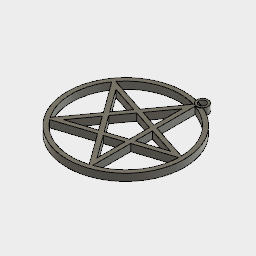
五角星挂件 v0 (Autodesk Fusion 360 design; units mm, degrees)
Autodesk Fusion 360 part; units mm, degrees
sketch "草图1" plane through (0, 0, 0) normal (0, 1, 0) x (1, 0, 0)
  circle A0 centre (70, -20) radius 40.6099
  line L0 (80.6872, 16.0595) -> (65.2067, -5.2476)
  line L1 (79.5492, 9.3893) -> (68.2067, -6.2223)
  line L2 (40.1586, 2.891) -> (65.2067, -5.2476)
  line L3 (45, -1.8364) -> (63.3525, -7.7995)
  line L4 (45, -1.8364) -> (56.3425, -17.448)
  line L5 (63.3525, -7.7995) -> (56.3425, -17.448)
  line L6 (54.4884, -20) -> (39.0079, -41.3071)
  line L7 (66.3525, -8.7743) -> (58.1966, -20)
  line L8 (56.3425, -22.552) -> (45, -38.1636)
  line L9 (39.0079, 1.3071) -> (54.4884, -20)
  line L10 (65.2067, -34.7524) -> (40.1586, -42.891)
  line L11 (56.3425, -22.552) -> (63.3525, -32.2005)
  line L12 (65.2067, -34.7524) -> (80.6872, -56.0595)
  line L13 (58.1966, -20) -> (66.3525, -31.2257)
  line L14 (68.2067, -33.7777) -> (79.5492, -49.3893)
  line L15 (63.3525, -32.2005) -> (45, -38.1636)
  line L16 (82.5492, -29.1175) -> (82.5492, -55.4545)
  line L17 (107.5972, -20.9789) -> (82.5492, -29.1175)
  line L18 (79.5492, -30.0923) -> (68.2067, -33.7777)
  line L19 (79.5492, -30.0923) -> (79.5492, -49.3893)
  line L20 (100.9017, -20) -> (82.5492, -25.9631)
  line L21 (79.5492, -26.9379) -> (66.3525, -31.2257)
  line L22 (82.5492, 15.4545) -> (82.5492, -10.8825)
  line L23 (82.5492, -14.0369) -> (82.5492, -25.9631)
  line L24 (66.3525, -8.7743) -> (79.5492, -13.0621)
  line L25 (82.5492, -14.0369) -> (100.9017, -20)
  line L26 (79.5492, 9.3893) -> (79.5492, -9.9077)
  line L27 (79.5492, -13.0621) -> (79.5492, -26.9379)
  line L28 (68.2067, -6.2223) -> (79.5492, -9.9077)
  line L29 (82.5492, -10.8825) -> (107.5972, -19.0211)
  circle A1 centre (70, -20) radius 37.6099
  point P0 (70, -20)
  dimension "d3" = 3
sketch "草图2" plane through (0, 0, 0) normal (0, 1, 0) x (1, 0, 0)
sketch "草图3" plane through (0, 0, 0) normal (0, 1, 0) x (1, 0, 0)
sketch "草图4" plane through (0, 0, 0) normal (0, 1, 0) x (1, 0, 0)
extrude "拉伸1" add sketch "草图1" along normal blind 5 contours A0 | L0 L2 L6 L9 L10 L12 L16 L17 L22 L29 A1 makes body 1
sketch "草图5" plane through (0, 0, 0) normal (0, 1, 0) x (1, 0, 0)
  circle A0 centre (10, -35) radius 4
  circle A1 centre (10, -35) radius 2.5
  dimension "d6" = 5
  measures "d6" diameter of A1
extrude "拉伸2" add sketch "草图5" along normal blind 5 separate body makes body 2
move_body "移动1" bodies 2 to x (1, 0, 0) y (0, 1, 0) z (0, 0, 1) at (73.4596, 0.2952, -54.7096)
combine "合并1" operation add target body 2 tool bodies 1
